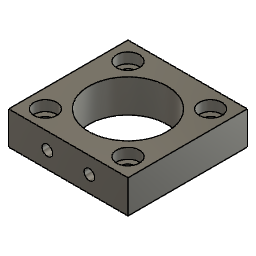
Nema8Mount v16 (Autodesk Fusion 360 archive; units mm, degrees)
design "Nema8Mount" references "tormach 770mx"
Autodesk Fusion 360 part; units mm, degrees
sketch "Sketch1" plane through (0, 0, 0) normal (0, 1, 0) x (1, 0, 0)
  line L0 (11.55, -11.55) -> (-11.55, -11.55)
  line L1 (-11.55, -11.55) -> (-11.55, 11.55)
  line L2 (-11.55, 11.55) -> (11.55, 11.55)
  line L3 (11.55, 11.55) -> (11.55, -11.55)
  line L4 (11.55, -11.55) -> (-11.55, 11.55) construction
  line L5 (-11.55, -11.55) -> (11.55, 11.55) construction
  dimension "d1" = 23.1
  dimension "d2" = 23.1
  constraint horizontal L0
  constraint perpendicular L0 L1
  constraint parallel L0 L2
  constraint parallel L1 L3
  constraint coincident L4 origin
  constraint coincident L5 origin
  measures "d1" distance of L1.end L2.end
  measures "d2" distance of L0.end L1.end
extrude "Extrude1" add sketch "Sketch1" along normal blind 6.4
sketch "Sketch2" plane through (0, 6.4, 0) normal (0, 1, 0) x (-1, 0, 0)
  line L0 (-11.55, -11.55) -> (11.55, -11.55)
  line L1 (11.55, -11.55) -> (11.55, 11.55)
  line L2 (11.55, 11.55) -> (-11.55, 11.55)
  line L3 (-11.55, 11.55) -> (-11.55, -11.55)
  line L4 (-8, 8) -> (8, 8) construction
  line L5 (8, 8) -> (8, -8) construction
  line L6 (8, -8) -> (-8, -8) construction
  line L7 (-8, -8) -> (-8, 8) construction
  line L8 (-8, 8) -> (8, -8) construction
  line L9 (8, 8) -> (-8, -8) construction
  circle A0 centre (0, 0) radius 7.6
  point P0 (8, -8)
  point P1 (-8, -8)
  point P2 (-8, 8)
  point P3 (8, 8)
  dimension "d5" = 16
  dimension "d6" = 16
  dimension "d7" = 15.2
  constraint horizontal L4
  constraint perpendicular L4 L5
  constraint parallel L4 L6
  constraint parallel L5 L7
  constraint coincident L8 A0.centre
  constraint coincident L9 A0.centre
  constraint coincident A0.centre origin
  constraint coincident P0 L5.end
  constraint coincident P1 L6.end
  constraint coincident P2 L4.start
  constraint coincident P3 L4.end
  measures "d5" distance of P0 P1
  measures "d6" distance of P3 P0
  measures "d7" diameter of A0
hole "Hole1" at (-8, 6.4, -8) direction (0, -1, 0) diameter 2.2 end through all counterbore diameter 4.4 counterbore depth 2
hole "Hole2" at (8, 6.4, -8) direction (0, -1, 0) diameter 2.2 end through all counterbore diameter 4.4 counterbore depth 2
hole "Hole3" at (8, 6.4, 8) direction (0, -1, 0) diameter 2.2 end through all counterbore diameter 4.4 counterbore depth 2
hole "Hole4" at (-8, 6.4, 8) direction (0, -1, 0) diameter 2.2 end through all counterbore diameter 4.4 counterbore depth 2
extrude "Extrude2" cut sketch "Sketch2" along normal through all and the other way through all contours A0
sketch "Sketch3" plane through (0, 0, 11.55) normal (0, 0, 1) x (1, 0, 0)
  line L0 (-11.55, 0) -> (11.55, 0)
  line L1 (11.55, 0) -> (11.55, 6.4)
  line L2 (11.55, 6.4) -> (-11.55, 6.4)
  line L3 (-11.55, 6.4) -> (-11.55, 0)
  line L4 (-11.55, 3.2) -> (11.55, 3.2) construction
  point P0 (-4.15, 3.2)
  point P1 (3.99, 3.2)
  dimension "d29" = 8.14
  dimension "d30" = 7.4
  constraint midpoint L3 L4.start
  constraint midpoint L1 L4.end
  constraint coincident L4 P0
  constraint coincident L4 P1
  measures "d29" distance of P0 P1
  measures "d30" distance of L3 P0
hole "Hole5" at (-4.07, 3.2, 11.55) direction (0, 0, -1) diameter 2.05 depth 7 tip angle 118
hole "Hole6" at (4.07, 3.2, 11.55) direction (0, 0, -1) diameter 2.05 depth 7 tip angle 118
